Autodesk Inventor part; units mm, degrees
(part 2 of 3)
  arc A17 (-11.8052, -4.5833) -> (-10.4532, -3.3962) centre (-11.8777, -3.1373) ccw
  arc A18 (-11.8052, -4.5833) -> (-10.4532, -3.3962) centre (-11.8777, -3.1373) ccw
  line L518 (-12.3915, -4.5833) -> (-11.8052, -4.5833)
  line L519 (-11.8052, -4.5833) -> (-12.3915, -4.5833)
  arc A19 (-13.2869, -3.5243) -> (-12.3915, -4.5833) centre (-12.3915, -3.6753) ccw
  arc A20 (-13.2869, -3.5243) -> (-12.3915, -4.5833) centre (-12.3915, -3.6753) ccw
  line L520 (10.764, -4.357) -> (10.8318, -4.3058)
  line L521 (10.8318, -4.3058) -> (10.764, -4.357)
  line L522 (10.6948, -4.4031) -> (10.764, -4.357)
  line L523 (10.764, -4.357) -> (10.6948, -4.4031)
  line L524 (10.6242, -4.4442) -> (10.6948, -4.4031)
  line L525 (10.6948, -4.4031) -> (10.6242, -4.4442)
  line L526 (10.5766, -4.468) -> (10.6242, -4.4442)
  line L527 (10.6242, -4.4442) -> (10.5766, -4.468)
  line L528 (10.4995, -4.5019) -> (10.5766, -4.468)
  line L529 (10.5766, -4.468) -> (10.4995, -4.5019)
  line L530 (10.4201, -4.5314) -> (10.4995, -4.5019)
  line L531 (10.4995, -4.5019) -> (10.4201, -4.5314)
  line L532 (10.3401, -4.5552) -> (10.4201, -4.5314)
  line L533 (10.4201, -4.5314) -> (10.3401, -4.5552)
  line L534 (10.2587, -4.574) -> (10.3401, -4.5552)
  line L535 (10.3401, -4.5552) -> (10.2587, -4.574)
  line L536 (10.1757, -4.5877) -> (10.2587, -4.574)
  line L537 (10.2587, -4.574) -> (10.1757, -4.5877)
  line L538 (10.0914, -4.5956) -> (10.1757, -4.5877)
  line L539 (10.1757, -4.5877) -> (10.0914, -4.5956)
  line L540 (10.0063, -4.5985) -> (10.0914, -4.5956)
  line L541 (10.0914, -4.5956) -> (10.0063, -4.5985)
  line L542 (9.9984, -4.5985) -> (10.0063, -4.5985)
  line L543 (10.0063, -4.5985) -> (9.9984, -4.5985)
  line L544 (9.9112, -4.5956) -> (9.9984, -4.5985)
  line L545 (9.9984, -4.5985) -> (9.9112, -4.5956)
  line L546 (9.8261, -4.5869) -> (9.9112, -4.5956)
  line L547 (9.9112, -4.5956) -> (9.8261, -4.5869)
  line L548 (9.7432, -4.5725) -> (9.8261, -4.5869)
  line L549 (9.8261, -4.5869) -> (9.7432, -4.5725)
  line L550 (9.6631, -4.5523) -> (9.7432, -4.5725)
  line L551 (9.7432, -4.5725) -> (9.6631, -4.5523)
  line L552 (9.5846, -4.5257) -> (9.6631, -4.5523)
  line L553 (9.6631, -4.5523) -> (9.5846, -4.5257)
  line L554 (9.5081, -4.4939) -> (9.5846, -4.5257)
  line L555 (9.5846, -4.5257) -> (9.5081, -4.4939)
  line L556 (9.4346, -4.4557) -> (9.5081, -4.4939)
  line L557 (9.5081, -4.4939) -> (9.4346, -4.4557)
  line L558 (9.4173, -4.4464) -> (9.4346, -4.4557)
  line L559 (9.4346, -4.4557) -> (9.4173, -4.4464)
  line L560 (9.3452, -4.4002) -> (9.4173, -4.4464)
  line L561 (9.4173, -4.4464) -> (9.3452, -4.4002)
  line L562 (9.2782, -4.3498) -> (9.3452, -4.4002)
  line L563 (9.3452, -4.4002) -> (9.2782, -4.3498)
  line L564 (9.2169, -4.2942) -> (9.2782, -4.3498)
  line L565 (9.2782, -4.3498) -> (9.2169, -4.2942)
  line L566 (9.1599, -4.2344) -> (9.2169, -4.2942)
  line L567 (9.2169, -4.2942) -> (9.1599, -4.2344)
  line L568 (9.1087, -4.1688) -> (9.1599, -4.2344)
  line L569 (9.1599, -4.2344) -> (9.1087, -4.1688)
  line L570 (9.0626, -4.0989) -> (9.1087, -4.1688)
  line L571 (9.1087, -4.1688) -> (9.0626, -4.0989)
  line L572 (9.0215, -4.0239) -> (9.0626, -4.0989)
  line L573 (9.0626, -4.0989) -> (9.0215, -4.0239)
  line L574 (9.0186, -4.0188) -> (9.0215, -4.0239)
  line L575 (9.0215, -4.0239) -> (9.0186, -4.0188)
  line L576 (8.9833, -3.9417) -> (9.0186, -4.0188)
  line L577 (9.0186, -4.0188) -> (8.9833, -3.9417)
  line L578 (8.953, -3.8631) -> (8.9833, -3.9417)
  line L579 (8.9833, -3.9417) -> (8.953, -3.8631)
  line L580 (8.9285, -3.7831) -> (8.953, -3.8631)
  line L581 (8.953, -3.8631) -> (8.9285, -3.7831)
  line L582 (8.909, -3.7023) -> (8.9285, -3.7831)
  line L583 (8.9285, -3.7831) -> (8.909, -3.7023)
  line L584 (8.8946, -3.6194) -> (8.909, -3.7023)
  line L585 (8.909, -3.7023) -> (8.8946, -3.6194)
  line L586 (8.886, -3.5351) -> (8.8946, -3.6194)
  line L587 (8.8946, -3.6194) -> (8.886, -3.5351)
  line L588 (8.8824, -3.45) -> (8.886, -3.5351)
  line L589 (8.886, -3.5351) -> (8.8824, -3.45)
  line L590 (8.8824, -3.4363) -> (8.8824, -3.45)
  line L591 (8.8824, -3.45) -> (8.8824, -3.4363)
  line L592 (8.8845, -3.3433) -> (8.8824, -3.4363)
  line L593 (8.8824, -3.4363) -> (8.8845, -3.3433)
  line L594 (8.8896, -3.2525) -> (8.8845, -3.3433)
  line L595 (8.8845, -3.3433) -> (8.8896, -3.2525)
  line L596 (8.8989, -3.1645) -> (8.8896, -3.2525)
  line L597 (8.8896, -3.2525) -> (8.8989, -3.1645)
  line L598 (8.9112, -3.0787) -> (8.8989, -3.1645)
  line L599 (8.8989, -3.1645) -> (8.9112, -3.0787)
  line L600 (8.9278, -2.9951) -> (8.9112, -3.0787)
  line L601 (8.9112, -3.0787) -> (8.9278, -2.9951)
  line L602 (8.9472, -2.9136) -> (8.9278, -2.9951)
  line L603 (8.9278, -2.9951) -> (8.9472, -2.9136)
  line L604 (8.971, -2.8343) -> (8.9472, -2.9136)
  line L605 (8.9472, -2.9136) -> (8.971, -2.8343)
  line L606 (8.9977, -2.7579) -> (8.971, -2.8343)
  line L607 (8.971, -2.8343) -> (8.9977, -2.7579)
  line L608 (9.0287, -2.6843) -> (8.9977, -2.7579)
  line L609 (8.9977, -2.7579) -> (9.0287, -2.6843)
  line L610 (9.0626, -2.6122) -> (9.0287, -2.6843)
  line L611 (9.0287, -2.6843) -> (9.0626, -2.6122)
  line L612 (9.1008, -2.543) -> (9.0626, -2.6122)
  line L613 (9.0626, -2.6122) -> (9.1008, -2.543)
  line L614 (9.1419, -2.476) -> (9.1008, -2.543)
  line L615 (9.1008, -2.543) -> (9.1419, -2.476)
  line L616 (9.1873, -2.4111) -> (9.1419, -2.476)
  line L617 (9.1419, -2.476) -> (9.1873, -2.4111)
  line L618 (9.2363, -2.3491) -> (9.1873, -2.4111)
  line L619 (9.1873, -2.4111) -> (9.2363, -2.3491)
  line L620 (9.2882, -2.2893) -> (9.2363, -2.3491)
  line L621 (9.2363, -2.3491) -> (9.2882, -2.2893)
  line L622 (9.2955, -2.2813) -> (9.2882, -2.2893)
  line L623 (9.2882, -2.2893) -> (9.2955, -2.2813)
  line L624 (9.3567, -2.2193) -> (9.2955, -2.2813)
  line L625 (9.2955, -2.2813) -> (9.3567, -2.2193)
  line L626 (9.4202, -2.1617) -> (9.3567, -2.2193)
  line L627 (9.3567, -2.2193) -> (9.4202, -2.1617)
  line L628 (9.4851, -2.109) -> (9.4202, -2.1617)
  line L629 (9.4202, -2.1617) -> (9.4851, -2.109)
  line L630 (9.5521, -2.0607) -> (9.4851, -2.109)
  line L631 (9.4851, -2.109) -> (9.5521, -2.0607)
  line L632 (9.6213, -2.0175) -> (9.5521, -2.0607)
  line L633 (9.5521, -2.0607) -> (9.6213, -2.0175)
  line L634 (9.692, -1.9785) -> (9.6213, -2.0175)
  line L635 (9.6213, -2.0175) -> (9.692, -1.9785)
  line L636 (9.7648, -1.9446) -> (9.692, -1.9785)
  line L637 (9.692, -1.9785) -> (9.7648, -1.9446)
  line L638 (9.8398, -1.9158) -> (9.7648, -1.9446)
  line L639 (9.7648, -1.9446) -> (9.8398, -1.9158)
  line L640 (9.9162, -1.8913) -> (9.8398, -1.9158)
  line L641 (9.8398, -1.9158) -> (9.9162, -1.8913)
  line L642 (9.9948, -1.8718) -> (9.9162, -1.8913)
  line L643 (9.9162, -1.8913) -> (9.9948, -1.8718)
  line L644 (10.0755, -1.8574) -> (9.9948, -1.8718)
  line L645 (9.9948, -1.8718) -> (10.0755, -1.8574)
  line L646 (10.1577, -1.8473) -> (10.0755, -1.8574)
  line L647 (10.0755, -1.8574) -> (10.1577, -1.8473)
  line L648 (10.2421, -1.8423) -> (10.1577, -1.8473)
  line L649 (10.1577, -1.8473) -> (10.2421, -1.8423)
  line L650 (10.2933, -1.8415) -> (10.2421, -1.8423)
  line L651 (10.2421, -1.8423) -> (10.2933, -1.8415)
  line L652 (10.3834, -1.8444) -> (10.2933, -1.8415)
  line L653 (10.2933, -1.8415) -> (10.3834, -1.8444)
  line L654 (10.4706, -1.8524) -> (10.3834, -1.8444)
  line L655 (10.3834, -1.8444) -> (10.4706, -1.8524)
  line L656 (10.5542, -1.8661) -> (10.4706, -1.8524)
  line L657 (10.4706, -1.8524) -> (10.5542, -1.8661)
  line L658 (10.635, -1.8855) -> (10.5542, -1.8661)
  line L659 (10.5542, -1.8661) -> (10.635, -1.8855)
  line L660 (10.7129, -1.91) -> (10.635, -1.8855)
  line L661 (10.635, -1.8855) -> (10.7129, -1.91)
  line L662 (10.7871, -1.9403) -> (10.7129, -1.91)
  line L663 (10.7129, -1.91) -> (10.7871, -1.9403)
  line L664 (10.8585, -1.9756) -> (10.7871, -1.9403)
  line L665 (10.7871, -1.9403) -> (10.8585, -1.9756)
  line L666 (10.927, -2.0167) -> (10.8585, -1.9756)
  line L667 (10.8585, -1.9756) -> (10.927, -2.0167)
  line L668 (10.9926, -2.0636) -> (10.927, -2.0167)
  line L669 (10.927, -2.0167) -> (10.9926, -2.0636)
  line L670 (11.0546, -2.1155) -> (10.9926, -2.0636)
  line L671 (10.9926, -2.0636) -> (11.0546, -2.1155)
  line L672 (11.1058, -2.1653) -> (11.0546, -2.1155)
  line L673 (11.0546, -2.1155) -> (11.1058, -2.1653)
  line L674 (11.1584, -2.2237) -> (11.1058, -2.1653)
  line L675 (11.1058, -2.1653) -> (11.1584, -2.2237)
  line L676 (11.206, -2.2857) -> (11.1584, -2.2237)
  line L677 (11.1584, -2.2237) -> (11.206, -2.2857)
  line L678 (11.2485, -2.3513) -> (11.206, -2.2857)
  line L679 (11.206, -2.2857) -> (11.2485, -2.3513)
  line L680 (11.286, -2.4198) -> (11.2485, -2.3513)
  line L681 (11.2485, -2.3513) -> (11.286, -2.4198)
  line L682 (11.3192, -2.4918) -> (11.286, -2.4198)
  line L683 (11.286, -2.4198) -> (11.3192, -2.4918)
  line L684 (11.348, -2.5675) -> (11.3192, -2.4918)
  line L685 (11.3192, -2.4918) -> (11.348, -2.5675)
  line L686 (11.3718, -2.6461) -> (11.348, -2.5675)
  line L687 (11.348, -2.5675) -> (11.3718, -2.6461)
  line L688 (11.3906, -2.7283) -> (11.3718, -2.6461)
  line L689 (11.3718, -2.6461) -> (11.3906, -2.7283)
  line L690 (11.4043, -2.8141) -> (11.3906, -2.7283)
  line L691 (11.3906, -2.7283) -> (11.4043, -2.8141)
  line L692 (11.4136, -2.9028) -> (11.4043, -2.8141)
  line L693 (11.4043, -2.8141) -> (11.4136, -2.9028)
  line L694 (11.418, -2.9951) -> (11.4136, -2.9028)
  line L695 (11.4136, -2.9028) -> (11.418, -2.9951)
  line L696 (11.4187, -3.0362) -> (11.418, -2.9951)
  line L697 (11.418, -2.9951) -> (11.4187, -3.0362)
  line L698 (11.4165, -3.1241) -> (11.4187, -3.0362)
  line L699 (11.4187, -3.0362) -> (11.4165, -3.1241)
  line L700 (11.4107, -3.2099) -> (11.4165, -3.1241)
  line L701 (11.4165, -3.1241) -> (11.4107, -3.2099)
  line L702 (11.3999, -3.2943) -> (11.4107, -3.2099)
  line L703 (11.4107, -3.2099) -> (11.3999, -3.2943)
  line L704 (11.3862, -3.3772) -> (11.3999, -3.2943)
  line L705 (11.3999, -3.2943) -> (11.3862, -3.3772)
  line L706 (11.3675, -3.4594) -> (11.3862, -3.3772)
  line L707 (11.3862, -3.3772) -> (11.3675, -3.4594)
  line L708 (11.3459, -3.5394) -> (11.3675, -3.4594)
  line L709 (11.3675, -3.4594) -> (11.3459, -3.5394)
  line L710 (11.3192, -3.618) -> (11.3459, -3.5394)
  line L711 (11.3459, -3.5394) -> (11.3192, -3.618)
  line L712 (11.2889, -3.6951) -> (11.3192, -3.618)
  line L713 (11.3192, -3.618) -> (11.2889, -3.6951)
  line L714 (11.2601, -3.7586) -> (11.2889, -3.6951)
  line L715 (11.2889, -3.6951) -> (11.2601, -3.7586)
  line L716 (11.2204, -3.8372) -> (11.2601, -3.7586)
  line L717 (11.2601, -3.7586) -> (11.2204, -3.8372)
  line L718 (11.1779, -3.9121) -> (11.2204, -3.8372)
  line L719 (11.2204, -3.8372) -> (11.1779, -3.9121)
  line L720 (11.1317, -3.9835) -> (11.1779, -3.9121)
  line L721 (11.1779, -3.9121) -> (11.1317, -3.9835)
  line L722 (11.082, -4.0513) -> (11.1317, -3.9835)
  line L723 (11.1317, -3.9835) -> (11.082, -4.0513)
  line L724 (11.0294, -4.1154) -> (11.082, -4.0513)
  line L725 (11.082, -4.0513) -> (11.0294, -4.1154)
  line L726 (10.9738, -4.176) -> (11.0294, -4.1154)
  line L727 (11.0294, -4.1154) -> (10.9738, -4.176)
  line L728 (10.9623, -4.1875) -> (10.9738, -4.176)
  line L729 (10.9738, -4.176) -> (10.9623, -4.1875)
  line L730 (10.8974, -4.2495) -> (10.9623, -4.1875)
  line L731 (10.9623, -4.1875) -> (10.8974, -4.2495)
  line L732 (10.8318, -4.3058) -> (10.8974, -4.2495)
  line L733 (10.8974, -4.2495) -> (10.8318, -4.3058)
  line L734 (-3.4143, -2.0689) -> (-3.8594, -4.5927)
  line L735 (-3.8594, -4.5927) -> (-3.4143, -2.0689)
  line L736 (-1.6963, -2.0689) -> (-3.4143, -2.0689)
  line L737 (-3.4143, -2.0689) -> (-1.6963, -2.0689)
  arc A21 (-1.4506, -3.3546) -> (-1.6963, -2.0689) centre (-1.726, -2.7409) ccw
  arc A22 (-1.4506, -3.3546) -> (-1.6963, -2.0689) centre (-1.726, -2.7409) ccw
  arc A23 (-1.2403, -3.7043) -> (-1.4506, -3.3546) centre (-2.0068, -3.9272) ccw
  arc A24 (-1.2403, -3.7043) -> (-1.4506, -3.3546) centre (-2.0068, -3.9272) ccw
  line L738 (-1.0022, -4.5927) -> (-1.2403, -3.7043)
  line L739 (-1.2403, -3.7043) -> (-1.0022, -4.5927)
  line L740 (-1.7842, -4.5927) -> (-1.0022, -4.5927)
  line L741 (-1.0022, -4.5927) -> (-1.7842, -4.5927)
  line L742 (-1.9465, -3.9869) -> (-1.7842, -4.5927)
  line L743 (-1.7842, -4.5927) -> (-1.9465, -3.9869)
  arc A25 (-1.9465, -3.9869) -> (-2.544, -3.5591) centre (-2.5929, -4.2585) ccw
  arc A26 (-1.9465, -3.9869) -> (-2.544, -3.5591) centre (-2.5929, -4.2585) ccw
  line L744 (-2.8935, -3.5591) -> (-2.544, -3.5591)
  line L745 (-2.544, -3.5591) -> (-2.8935, -3.5591)
  line L746 (-3.0757, -4.5927) -> (-2.8935, -3.5591)
  line L747 (-2.8935, -3.5591) -> (-3.0757, -4.5927)
  line L748 (-3.8594, -4.5927) -> (-3.0757, -4.5927)
  line L749 (-3.0757, -4.5927) -> (-3.8594, -4.5927)
  line L750 (-9.2507, -2.0595) -> (-10.0381, -2.0595)
  line L751 (-10.0381, -2.0595) -> (-9.2507, -2.0595)
  line L752 (-9.134, -3.7743) -> (-9.2507, -2.0595)
  line L753 (-9.2507, -2.0595) -> (-9.134, -3.7743)
  line L754 (-8.4342, -2.0595) -> (-9.134, -3.7743)
  spline S0 degree 3 poles (0.7832, -2.4934) (0.8407, -2.4926) (0.8976, -2.5061) (1.0487, -2.5614) (1.1497, -2.6172) (1.3156, -2.7342) (1.3817, -2.7882) (1.4417, -2.8447) knots 4.484634 4.484634 4.484634 4.484634 4.865969 4.865969 5.478673 5.478673 5.90022 5.90022 5.90022 5.90022
  line L755 (0.7832, -2.4934) -> (0.8407, -2.4926) construction
  line L756 (0.8407, -2.4926) -> (0.8976, -2.5061) construction
  line L757 (0.8976, -2.5061) -> (1.0487, -2.5614) construction
  line L758 (1.0487, -2.5614) -> (1.1497, -2.6172) construction
  line L759 (1.1497, -2.6172) -> (1.3156, -2.7342) construction
  line L760 (1.3156, -2.7342) -> (1.3817, -2.7882) construction
  line L761 (1.3817, -2.7882) -> (1.4417, -2.8447) construction
  line L762 (-9.134, -3.7743) -> (-8.4342, -2.0595)
  spline S1 degree 3 poles (1.4417, -2.8447) (1.3817, -2.7882) (1.3156, -2.7342) (1.1497, -2.6172) (1.0487, -2.5614) (0.8976, -2.5061) (0.8407, -2.4926) (0.7832, -2.4934) knots -5.90022 -5.90022 -5.90022 -5.90022 -5.478673 -5.478673 -4.865969 -4.865969 -4.484634 -4.484634 -4.484634 -4.484634
  line L763 (1.4417, -2.8447) -> (1.3817, -2.7882) construction
  line L764 (1.3817, -2.7882) -> (1.3156, -2.7342) construction
  line L765 (1.3156, -2.7342) -> (1.1497, -2.6172) construction
  line L766 (1.1497, -2.6172) -> (1.0487, -2.5614) construction
  line L767 (1.0487, -2.5614) -> (0.8976, -2.5061) construction
  line L768 (0.8976, -2.5061) -> (0.8407, -2.4926) construction
  line L769 (0.8407, -2.4926) -> (0.7832, -2.4934) construction
  line L770 (-8.0608, -2.0595) -> (-8.4342, -2.0595)
  line L771 (-8.4342, -2.0595) -> (-8.0608, -2.0595)
  line L772 (-7.8698, -3.7104) -> (-8.0608, -2.0595)
  line L773 (-8.0608, -2.0595) -> (-7.8698, -3.7104)
  line L774 (-7.1961, -2.0595) -> (-7.8698, -3.7104)
  line L775 (-7.8698, -3.7104) -> (-7.1961, -2.0595)
  line L776 (-6.4191, -2.0595) -> (-7.1961, -2.0595)
  line L777 (-7.1961, -2.0595) -> (-6.4191, -2.0595)
  line L778 (-7.7213, -4.5833) -> (-6.4191, -2.0595)
  line L779 (-6.4191, -2.0595) -> (-7.7213, -4.5833)
  line L780 (-8.1744, -4.5833) -> (-7.7213, -4.5833)
  line L781 (-7.7213, -4.5833) -> (-8.1744, -4.5833)
  line L782 (-8.4008, -2.9217) -> (-8.1744, -4.5833)
  line L783 (-8.1744, -4.5833) -> (-8.4008, -2.9217)
  line L784 (-9.1859, -4.5833) -> (-8.4008, -2.9217)
  line L785 (-8.4008, -2.9217) -> (-9.1859, -4.5833)
  line L786 (-9.626, -4.5833) -> (-9.1859, -4.5833)
  line L787 (-9.1859, -4.5833) -> (-9.626, -4.5833)
  line L788 (-10.0381, -2.0595) -> (-9.626, -4.5833)
  line L789 (-9.626, -4.5833) -> (-10.0381, -2.0595)
  line L790 (6.6315, -3.3693) -> (7.0461, -3.3693)
  line L791 (7.0461, -3.3693) -> (6.6315, -3.3693)
  line L792 (6.385, -4.5531) -> (6.6315, -3.3693)
  line L793 (6.6315, -3.3693) -> (6.385, -4.5531)
  line L794 (6.0281, -4.5531) -> (6.385, -4.5531)
  line L795 (6.385, -4.5531) -> (6.0281, -4.5531)
  line L796 (6.5861, -1.887) -> (6.0281, -4.5531)
  line L797 (6.0281, -4.5531) -> (6.5861, -1.887)
  line L798 (7.7043, -1.887) -> (6.5861, -1.887)
  line L799 (6.5861, -1.887) -> (7.7043, -1.887)
  line L800 (7.811, -1.8884) -> (7.7043, -1.887)
  line L801 (7.7043, -1.887) -> (7.811, -1.8884)
  line L802 (7.9083, -1.8927) -> (7.811, -1.8884)
  line L803 (7.811, -1.8884) -> (7.9083, -1.8927)
  line L804 (7.9963, -1.9007) -> (7.9083, -1.8927)
  line L805 (7.9083, -1.8927) -> (7.9963, -1.9007)
  line L806 (8.0756, -1.9115) -> (7.9963, -1.9007)
  line L807 (7.9963, -1.9007) -> (8.0756, -1.9115)
  line L808 (8.1463, -1.9252) -> (8.0756, -1.9115)
  line L809 (8.0756, -1.9115) -> (8.1463, -1.9252)
  line L810 (8.2061, -1.941) -> (8.1463, -1.9252)
  line L811 (8.1463, -1.9252) -> (8.2061, -1.941)
  line L812 (8.284, -1.9742) -> (8.2061, -1.941)
  line L813 (8.2061, -1.941) -> (8.284, -1.9742)
  line L814 (8.3532, -2.0175) -> (8.284, -1.9742)
  line L815 (8.284, -1.9742) -> (8.3532, -2.0175)
  line L816 (8.4145, -2.0723) -> (8.3532, -2.0175)
  line L817 (8.3532, -2.0175) -> (8.4145, -2.0723)
  line L818 (8.4671, -2.1386) -> (8.4145, -2.0723)
  line L819 (8.4145, -2.0723) -> (8.4671, -2.1386)
  line L820 (8.475, -2.1508) -> (8.4671, -2.1386)
  line L821 (8.4671, -2.1386) -> (8.475, -2.1508)
  line L822 (8.5111, -2.2179) -> (8.475, -2.1508)
  line L823 (8.475, -2.1508) -> (8.5111, -2.2179)
  line L824 (8.5392, -2.2921) -> (8.5111, -2.2179)
  line L825 (8.5111, -2.2179) -> (8.5392, -2.2921)
  line L826 (8.5579, -2.3729) -> (8.5392, -2.2921)
  line L827 (8.5392, -2.2921) -> (8.5579, -2.3729)
  line L828 (8.5687, -2.4608) -> (8.5579, -2.3729)
  line L829 (8.5579, -2.3729) -> (8.5687, -2.4608)
  line L830 (8.5716, -2.5358) -> (8.5687, -2.4608)
  line L831 (8.5687, -2.4608) -> (8.5716, -2.5358)
  line L832 (8.5673, -2.6245) -> (8.5716, -2.5358)
  line L833 (8.5716, -2.5358) -> (8.5673, -2.6245)
  line L834 (8.555, -2.7089) -> (8.5673, -2.6245)
  line L835 (8.5673, -2.6245) -> (8.555, -2.7089)
  line L836 (8.5349, -2.7882) -> (8.555, -2.7089)
  line L837 (8.555, -2.7089) -> (8.5349, -2.7882)
  line L838 (8.506, -2.8639) -> (8.5349, -2.7882)
  line L839 (8.5349, -2.7882) -> (8.506, -2.8639)
  line L840 (8.4685, -2.9352) -> (8.506, -2.8639)
  line L841 (8.506, -2.8639) -> (8.4685, -2.9352)
  line L842 (8.4238, -3.0023) -> (8.4685, -2.9352)
  line L843 (8.4685, -2.9352) -> (8.4238, -3.0023)
  line L844 (8.3698, -3.065) -> (8.4238, -3.0023)
  line L845 (8.4238, -3.0023) -> (8.3698, -3.065)
  line L846 (8.3589, -3.0765) -> (8.3698, -3.065)
  line L847 (8.3698, -3.065) -> (8.3589, -3.0765)
  line L848 (8.3085, -3.122) -> (8.3589, -3.0765)
  line L849 (8.3589, -3.0765) -> (8.3085, -3.122)
  line L850 (8.2515, -3.1638) -> (8.3085, -3.122)
  line L851 (8.3085, -3.122) -> (8.2515, -3.1638)
  line L852 (8.1888, -3.2027) -> (8.2515, -3.1638)
  line L853 (8.2515, -3.1638) -> (8.1888, -3.2027)
  line L854 (8.1189, -3.2373) -> (8.1888, -3.2027)
  line L855 (8.1888, -3.2027) -> (8.1189, -3.2373)
  line L856 (8.0432, -3.2676) -> (8.1189, -3.2373)
  line L857 (8.1189, -3.2373) -> (8.0432, -3.2676)
  line L858 (7.9602, -3.295) -> (8.0432, -3.2676)
  line L859 (8.0432, -3.2676) -> (7.9602, -3.295)
  line L860 (7.8716, -3.3188) -> (7.9602, -3.295)
  line L861 (7.9602, -3.295) -> (7.8716, -3.3188)
  line L862 (7.7764, -3.3383) -> (7.8716, -3.3188)
  line L863 (7.8716, -3.3188) -> (7.7764, -3.3383)
  line L864 (7.674, -3.3541) -> (7.7764, -3.3383)
  line L865 (7.7764, -3.3383) -> (7.674, -3.3541)
  line L866 (7.6719, -3.3548) -> (7.674, -3.3541)
  line L867 (7.674, -3.3541) -> (7.6719, -3.3548)
  line L868 (7.7468, -3.414) -> (7.6719, -3.3548)
  line L869 (7.6719, -3.3548) -> (7.7468, -3.414)
  line L870 (7.811, -3.4723) -> (7.7468, -3.414)
  line L871 (7.7468, -3.414) -> (7.811, -3.4723)
  line L872 (7.8644, -3.5307) -> (7.811, -3.4723)
  line L873 (7.811, -3.4723) -> (7.8644, -3.5307)
  line L874 (7.8918, -3.5654) -> (7.8644, -3.5307)
  line L875 (7.8644, -3.5307) -> (7.8918, -3.5654)
  line L876 (7.9415, -3.6374) -> (7.8918, -3.5654)
  line L877 (7.8918, -3.5654) -> (7.9415, -3.6374)
  line L878 (7.9876, -3.7103) -> (7.9415, -3.6374)
  line L879 (7.9415, -3.6374) -> (7.9876, -3.7103)
  line L880 (8.0309, -3.7838) -> (7.9876, -3.7103)
  line L881 (7.9876, -3.7103) -> (8.0309, -3.7838)
  line L882 (8.0713, -3.8581) -> (8.0309, -3.7838)
  line L883 (8.0309, -3.7838) -> (8.0713, -3.8581)
  line L884 (8.1088, -3.933) -> (8.0713, -3.8581)
  line L885 (8.0713, -3.8581) -> (8.1088, -3.933)
  line L886 (8.1434, -4.0087) -> (8.1088, -3.933)
  line L887 (8.1088, -3.933) -> (8.1434, -4.0087)
  line L888 (8.1607, -4.0513) -> (8.1434, -4.0087)
  line L889 (8.1434, -4.0087) -> (8.1607, -4.0513)
  line L890 (8.3647, -4.5531) -> (8.1607, -4.0513)
  line L891 (8.1607, -4.0513) -> (8.3647, -4.5531)
  line L892 (7.966, -4.5531) -> (8.3647, -4.5531)
  line L893 (8.3647, -4.5531) -> (7.966, -4.5531)
  line L894 (7.7757, -4.057) -> (7.966, -4.5531)
  line L895 (7.966, -4.5531) -> (7.7757, -4.057)
  line L896 (7.7411, -3.9712) -> (7.7757, -4.057)
  line L897 (7.7757, -4.057) -> (7.7411, -3.9712)
  line L898 (7.705, -3.8898) -> (7.7411, -3.9712)
  line L899 (7.7411, -3.9712) -> (7.705, -3.8898)
  line L900 (7.6675, -3.8119) -> (7.705, -3.8898)
  line L901 (7.705, -3.8898) -> (7.6675, -3.8119)
  line L902 (7.6286, -3.7377) -> (7.6675, -3.8119)
  line L903 (7.6675, -3.8119) -> (7.6286, -3.7377)
  line L904 (7.5882, -3.6677) -> (7.6286, -3.7377)
  line L905 (7.6286, -3.7377) -> (7.5882, -3.6677)
  line L906 (7.5457, -3.6014) -> (7.5882, -3.6677)
  line L907 (7.5882, -3.6677) -> (7.5457, -3.6014)
  line L908 (7.5392, -3.5913) -> (7.5457, -3.6014)
  line L909 (7.5457, -3.6014) -> (7.5392, -3.5913)
  line L910 (7.4801, -3.5127) -> (7.5392, -3.5913)
  line L911 (7.5392, -3.5913) -> (7.4801, -3.5127)
  line L912 (7.421, -3.4543) -> (7.4801, -3.5127)
  line L913 (7.4801, -3.5127) -> (7.421, -3.4543)
  line L914 (7.3604, -3.4147) -> (7.421, -3.4543)
  line L915 (7.421, -3.4543) -> (7.3604, -3.4147)
  line L916 (7.3539, -3.4111) -> (7.3604, -3.4147)
  line L917 (7.3604, -3.4147) -> (7.3539, -3.4111)
  line L918 (7.2934, -3.3916) -> (7.3539, -3.4111)
  line L919 (7.3539, -3.4111) -> (7.2934, -3.3916)
  line L920 (7.2162, -3.3779) -> (7.2934, -3.3916)
  line L921 (7.2934, -3.3916) -> (7.2162, -3.3779)
  line L922 (7.1218, -3.3707) -> (7.2162, -3.3779)
  line L923 (7.2162, -3.3779) -> (7.1218, -3.3707)
  line L924 (7.0461, -3.3693) -> (7.1218, -3.3707)
  line L925 (7.1218, -3.3707) -> (7.0461, -3.3693)
  line L926 (-3.9191, -2.0689) -> (-5.9191, -2.0689)
  line L927 (-5.9191, -2.0689) -> (-3.9191, -2.0689)
  line L928 (-3.994, -2.4934) -> (-3.9191, -2.0689)
  line L929 (-3.9191, -2.0689) -> (-3.994, -2.4934)
  line L930 (-5.202, -2.4934) -> (-3.994, -2.4934)
  line L931 (-3.994, -2.4934) -> (-5.202, -2.4934)
  line L932 (-5.3149, -3.1336) -> (-5.202, -2.4934)
  line L933 (-5.202, -2.4934) -> (-5.3149, -3.1336)
  line L934 (-4.2021, -3.1336) -> (-5.3149, -3.1336)
  line L935 (-5.3149, -3.1336) -> (-4.2021, -3.1336)
  line L936 (-4.2717, -3.5281) -> (-4.2021, -3.1336)
  line L937 (-4.2021, -3.1336) -> (-4.2717, -3.5281)
  line L938 (-5.3845, -3.5281) -> (-4.2717, -3.5281)
  line L939 (-4.2717, -3.5281) -> (-5.3845, -3.5281)
  line L940 (-5.4974, -4.1682) -> (-5.3845, -3.5281)
  line L941 (-5.3845, -3.5281) -> (-5.4974, -4.1682)
  line L942 (-4.2893, -4.1682) -> (-5.4974, -4.1682)
  line L943 (-5.4974, -4.1682) -> (-4.2893, -4.1682)
  line L944 (-4.3642, -4.5927) -> (-4.2893, -4.1682)
  line L945 (-4.2893, -4.1682) -> (-4.3642, -4.5927)
  line L946 (-6.3642, -4.5927) -> (-4.3642, -4.5927)
  line L947 (-4.3642, -4.5927) -> (-6.3642, -4.5927)
  line L948 (-5.9191, -2.0689) -> (-6.3642, -4.5927)
  line L949 (-6.3642, -4.5927) -> (-5.9191, -2.0689)
  line L950 (16.3572, -3.2784) -> (16.4235, -3.2243)
  line L951 (16.4235, -3.2243) -> (16.3572, -3.2784)
  line L952 (16.2916, -3.3209) -> (16.3572, -3.2784)
  line L953 (16.3572, -3.2784) -> (16.2916, -3.3209)
  line L954 (16.2801, -3.3274) -> (16.2916, -3.3209)
  line L955 (16.2916, -3.3209) -> (16.2801, -3.3274)
  line L956 (16.2037, -3.3635) -> (16.2801, -3.3274)
  line L957 (16.2801, -3.3274) -> (16.2037, -3.3635)
  line L958 (16.1243, -3.3923) -> (16.2037, -3.3635)
  line L959 (16.2037, -3.3635) -> (16.1243, -3.3923)
  line L960 (16.0544, -3.4111) -> (16.1243, -3.3923)
  line L961 (16.1243, -3.3923) -> (16.0544, -3.4111)
  line L962 (15.9708, -3.4291) -> (16.0544, -3.4111)
  line L963 (16.0544, -3.4111) -> (15.9708, -3.4291)
  line L964 (15.8872, -3.4435) -> (15.9708, -3.4291)
  line L965 (15.9708, -3.4291) -> (15.8872, -3.4435)
  line L966 (15.8035, -3.455) -> (15.8872, -3.4435)
  line L967 (15.8872, -3.4435) -> (15.8035, -3.455)
  line L968 (15.7192, -3.4637) -> (15.8035, -3.455)
  line L969 (15.8035, -3.455) -> (15.7192, -3.4637)
  line L970 (15.6348, -3.4687) -> (15.7192, -3.4637)
  line L971 (15.7192, -3.4637) -> (15.6348, -3.4687)
  line L972 (15.5497, -3.4709) -> (15.6348, -3.4687)
  line L973 (15.6348, -3.4687) -> (15.5497, -3.4709)
  line L974 (14.8692, -3.4709) -> (15.5497, -3.4709)
  line L975 (15.5497, -3.4709) -> (14.8692, -3.4709)
  line L976 (14.6435, -4.5531) -> (14.8692, -3.4709)
  line L977 (14.8692, -3.4709) -> (14.6435, -4.5531)
  line L978 (14.2874, -4.5531) -> (14.6435, -4.5531)
  line L979 (14.6435, -4.5531) -> (14.2874, -4.5531)
  line L980 (14.8454, -1.887) -> (14.2874, -4.5531)
  line L981 (14.2874, -4.5531) -> (14.8454, -1.887)
  line L982 (15.9578, -1.887) -> (14.8454, -1.887)
  line L983 (14.8454, -1.887) -> (15.9578, -1.887)
  line L984 (16.0631, -1.8891) -> (15.9578, -1.887)
  line L985 (15.9578, -1.887) -> (16.0631, -1.8891)
  line L986 (16.1575, -1.8963) -> (16.0631, -1.8891)
  line L987 (16.0631, -1.8891) -> (16.1575, -1.8963)
  line L988 (16.2419, -1.9086) -> (16.1575, -1.8963)
  line L989 (16.1575, -1.8963) -> (16.2419, -1.9086)
  line L990 (16.3154, -1.9252) -> (16.2419, -1.9086)
  line L991 (16.2419, -1.9086) -> (16.3154, -1.9252)
  line L992 (16.3788, -1.9468) -> (16.3154, -1.9252)
  line L993 (16.3154, -1.9252) -> (16.3788, -1.9468)
  line L994 (16.3925, -1.9526) -> (16.3788, -1.9468)
  line L995 (16.3788, -1.9468) -> (16.3925, -1.9526)
  line L996 (16.461, -1.9922) -> (16.3925, -1.9526)
  line L997 (16.3925, -1.9526) -> (16.461, -1.9922)
  line L998 (16.5245, -2.0434) -> (16.461, -1.9922)
  line L999 (16.461, -1.9922) -> (16.5245, -2.0434)
  line L1000 (16.5807, -2.1061) -> (16.5245, -2.0434)
  line L1001 (16.5245, -2.0434) -> (16.5807, -2.1061)
  line L1002 (16.6305, -2.1797) -> (16.5807, -2.1061)
  line L1003 (16.5807, -2.1061) -> (16.6305, -2.1797)
  line L1004 (16.6679, -2.2532) -> (16.6305, -2.1797)
  line L1005 (16.6305, -2.1797) -> (16.6679, -2.2532)
  line L1006 (16.6961, -2.3311) -> (16.6679, -2.2532)
  line L1007 (16.6679, -2.2532) -> (16.6961, -2.3311)
  line L1008 (16.7148, -2.4125) -> (16.6961, -2.3311)
  line L1009 (16.6961, -2.3311) -> (16.7148, -2.4125)
  line L1010 (16.7242, -2.4976) -> (16.7148, -2.4125)
  line L1011 (16.7148, -2.4125) -> (16.7242, -2.4976)
  line L1012 (16.7249, -2.5416) -> (16.7242, -2.4976)
  line L1013 (16.7242, -2.4976) -> (16.7249, -2.5416)
  line L1014 (16.7213, -2.6231) -> (16.7249, -2.5416)
  line L1015 (16.7249, -2.5416) -> (16.7213, -2.6231)
  line L1016 (16.709, -2.7053) -> (16.7213, -2.6231)
  line L1017 (16.7213, -2.6231) -> (16.709, -2.7053)
  line L1018 (16.6889, -2.7882) -> (16.709, -2.7053)
  line L1019 (16.709, -2.7053) -> (16.6889, -2.7882)
  line L1020 (16.6607, -2.8718) -> (16.6889, -2.7882)
  line L1021 (16.6889, -2.7882) -> (16.6607, -2.8718)
  line L1022 (16.6579, -2.8783) -> (16.6607, -2.8718)
  line L1023 (16.6607, -2.8718) -> (16.6579, -2.8783)
  line L1024 (16.6211, -2.9619) -> (16.6579, -2.8783)
  line L1025 (16.6579, -2.8783) -> (16.6211, -2.9619)
  line L1026 (16.58, -3.0376) -> (16.6211, -2.9619)
  line L1027 (16.6211, -2.9619) -> (16.58, -3.0376)
  line L1028 (16.5338, -3.1054) -> (16.58, -3.0376)
  line L1029 (16.58, -3.0376) -> (16.5338, -3.1054)
  line L1030 (16.4891, -3.1602) -> (16.5338, -3.1054)
  line L1031 (16.5338, -3.1054) -> (16.4891, -3.1602)
  line L1032 (16.4235, -3.2243) -> (16.4891, -3.1602)
  line L1033 (16.4891, -3.1602) -> (16.4235, -3.2243)
  line L1034 (0.1973, -4.5927) -> (0.6148, -4.5927)
  line L1035 (0.6148, -4.5927) -> (0.1973, -4.5927)
  arc A27 (-0.5477, -4.4051) -> (0.1973, -4.5927) centre (0.1995, -3.0111) ccw
  arc A28 (-0.5477, -4.4051) -> (0.1973, -4.5927) centre (0.1995, -3.0111) ccw
  line L1036 (-0.4491, -3.846) -> (-0.5477, -4.4051)
  line L1037 (-0.5477, -4.4051) -> (-0.4491, -3.846)
  arc A29 (-0.4491, -3.846) -> (0.221, -4.1475) centre (1.0231, -1.4694) ccw
  arc A30 (-0.4491, -3.846) -> (0.221, -4.1475) centre (1.0231, -1.4694) ccw
  spline S2 degree 3 poles (0.3525, -4.1684) (0.3082, -4.1688) (0.2647, -4.1605) (0.221, -4.1475) knots 5.607238 5.607238 5.607238 5.607238 5.899629 5.899629 5.899629 5.899629
  line L1038 (0.3525, -4.1684) -> (0.3082, -4.1688) construction
  line L1039 (0.3082, -4.1688) -> (0.2647, -4.1605) construction
  line L1040 (0.2647, -4.1605) -> (0.221, -4.1475) construction
  spline S3 degree 3 poles (0.221, -4.1475) (0.2647, -4.1605) (0.3082, -4.1688) (0.3525, -4.1684) knots -5.899629 -5.899629 -5.899629 -5.899629 -5.607238 -5.607238 -5.607238 -5.607238
  line L1041 (0.221, -4.1475) -> (0.2647, -4.1605) construction
  line L1042 (0.2647, -4.1605) -> (0.3082, -4.1688) construction
  line L1043 (0.3082, -4.1688) -> (0.3525, -4.1684) construction
  arc A31 (0.3525, -4.1684) -> (0.4849, -3.582) centre (0.3521, -3.8601) ccw
  arc A32 (0.3525, -4.1684) -> (0.4849, -3.582) centre (0.3521, -3.8601) ccw
  line L1044 (0.0726, -3.3754) -> (0.4849, -3.582)
  line L1045 (0.4849, -3.582) -> (0.0726, -3.3754)
  arc A33 (-0.2619, -2.715) -> (0.0726, -3.3754) centre (0.3342, -2.828) ccw
  arc A34 (-0.2619, -2.715) -> (0.0726, -3.3754) centre (0.3342, -2.828) ccw
  arc A35 (0.5213, -2.0689) -> (-0.2619, -2.715) centre (0.5213, -2.8666) ccw
  arc A36 (0.5213, -2.0689) -> (-0.2619, -2.715) centre (0.5213, -2.8666) ccw
  line L1046 (0.7868, -2.0689) -> (0.5213, -2.0689)
  line L1047 (0.5213, -2.0689) -> (0.7868, -2.0689)
  arc A37 (0.7935, -2.0689) -> (0.7868, -2.0689) centre (0.7982, -3.6505) ccw
  arc A38 (0.7935, -2.0689) -> (0.7868, -2.0689) centre (0.7982, -3.6505) ccw
  line L1048 (0.8097, -2.0689) -> (0.7935, -2.0689)
  line L1049 (0.7935, -2.0689) -> (0.8097, -2.0689)
  arc A39 (1.5455, -2.2565) -> (0.8097, -2.0689) centre (0.7982, -3.6505) ccw
  arc A40 (1.5455, -2.2565) -> (0.8097, -2.0689) centre (0.7982, -3.6505) ccw
  line L1050 (1.4417, -2.8447) -> (1.5455, -2.2565)
  line L1051 (1.5455, -2.2565) -> (1.4417, -2.8447)
  arc A41 (0.7832, -2.4934) -> (0.6511, -3.0796) centre (0.8036, -2.806) ccw
  arc A42 (0.7832, -2.4934) -> (0.6511, -3.0796) centre (0.8036, -2.806) ccw
  line L1052 (1.0669, -3.2879) -> (0.6511, -3.0796)
  line L1053 (0.6511, -3.0796) -> (1.0669, -3.2879)
  arc A43 (1.3891, -3.9863) -> (1.0669, -3.2879) centre (0.7759, -3.8457) ccw
  arc A44 (1.3891, -3.9863) -> (1.0669, -3.2879) centre (0.7759, -3.8457) ccw
  arc A45 (0.6148, -4.5927) -> (1.3891, -3.9863) centre (0.6148, -3.795) ccw
  arc A46 (0.6148, -4.5927) -> (1.3891, -3.9863) centre (0.6148, -3.795) ccw
  line L1054 (12.1908, -3.5257) -> (12.5333, -1.887)
  line L1055 (12.5333, -1.887) -> (12.1908, -3.5257)
  line L1056 (12.1713, -3.631) -> (12.1908, -3.5257)
  line L1057 (12.1908, -3.5257) -> (12.1713, -3.631)
  line L1058 (12.1577, -3.7196) -> (12.1713, -3.631)
  line L1059 (12.1713, -3.631) -> (12.1577, -3.7196)
  line L1060 (12.1504, -3.7925) -> (12.1577, -3.7196)
  line L1061 (12.1577, -3.7196) -> (12.1504, -3.7925)
  line L1062 (12.149, -3.8278) -> (12.1504, -3.7925)
  line L1063 (12.1504, -3.7925) -> (12.149, -3.8278)
  line L1064 (12.1562, -3.9121) -> (12.149, -3.8278)
  line L1065 (12.149, -3.8278) -> (12.1562, -3.9121)
  line L1066 (12.1778, -3.99) -> (12.1562, -3.9121)
  line L1067 (12.1562, -3.9121) -> (12.1778, -3.99)
  line L1068 (12.2139, -4.0606) -> (12.1778, -3.99)
  line L1069 (12.1778, -3.99) -> (12.2139, -4.0606)
  line L1070 (12.2636, -4.1241) -> (12.2139, -4.0606)
  line L1071 (12.2139, -4.0606) -> (12.2636, -4.1241)
  line L1072 (12.3184, -4.1731) -> (12.2636, -4.1241)
  line L1073 (12.2636, -4.1241) -> (12.3184, -4.1731)
  line L1074 (12.3833, -4.2171) -> (12.3184, -4.1731)
  line L1075 (12.3184, -4.1731) -> (12.3833, -4.2171)
  line L1076 (12.4547, -4.2517) -> (12.3833, -4.2171)
  line L1077 (12.3833, -4.2171) -> (12.4547, -4.2517)
  line L1078 (12.5318, -4.2777) -> (12.4547, -4.2517)
  line L1079 (12.4547, -4.2517) -> (12.5318, -4.2777)
  line L1080 (12.6147, -4.295) -> (12.5318, -4.2777)
  line L1081 (12.5318, -4.2777) -> (12.6147, -4.295)
  line L1082 (12.7041, -4.3036) -> (12.6147, -4.295)
  line L1083 (12.6147, -4.295) -> (12.7041, -4.3036)
  line L1084 (12.7438, -4.3043) -> (12.7041, -4.3036)
  line L1085 (12.7041, -4.3036) -> (12.7438, -4.3043)
  line L1086 (12.8296, -4.3) -> (12.7438, -4.3043)
  line L1087 (12.7438, -4.3043) -> (12.8296, -4.3)
  line L1088 (12.9125, -4.287) -> (12.8296, -4.3)
  line L1089 (12.8296, -4.3) -> (12.9125, -4.287)
  line L1090 (12.9925, -4.2654) -> (12.9125, -4.287)
  line L1091 (12.9125, -4.287) -> (12.9925, -4.2654)
  line L1092 (13.0711, -4.2358) -> (12.9925, -4.2654)
  line L1093 (12.9925, -4.2654) -> (13.0711, -4.2358)
  line L1094 (13.1237, -4.2099) -> (13.0711, -4.2358)
  line L1095 (13.0711, -4.2358) -> (13.1237, -4.2099)
  line L1096 (13.1944, -4.1659) -> (13.1237, -4.2099)
  line L1097 (13.1237, -4.2099) -> (13.1944, -4.1659)
  line L1098 (13.2593, -4.1147) -> (13.1944, -4.1659)
  line L1099 (13.1944, -4.1659) -> (13.2593, -4.1147)
  line L1100 (13.3169, -4.0549) -> (13.2593, -4.1147)
  line L1101 (13.2593, -4.1147) -> (13.3169, -4.0549)
  line L1102 (13.3681, -3.9878) -> (13.3169, -4.0549)
  line L1103 (13.3169, -4.0549) -> (13.3681, -3.9878)
  line L1104 (13.3999, -3.9352) -> (13.3681, -3.9878)
  line L1105 (13.3681, -3.9878) -> (13.3999, -3.9352)
  line L1106 (13.428, -3.8804) -> (13.3999, -3.9352)
  line L1107 (13.3999, -3.9352) -> (13.428, -3.8804)
  line L1108 (13.4554, -3.817) -> (13.428, -3.8804)
  line L1109 (13.428, -3.8804) -> (13.4554, -3.817)
  line L1110 (13.4813, -3.7456) -> (13.4554, -3.817)
  line L1111 (13.4554, -3.817) -> (13.4813, -3.7456)
  line L1112 (13.5073, -3.6663) -> (13.4813, -3.7456)
  line L1113 (13.4813, -3.7456) -> (13.5073, -3.6663)
  line L1114 (13.5318, -3.5783) -> (13.5073, -3.6663)
  line L1115 (13.5073, -3.6663) -> (13.5318, -3.5783)
  line L1116 (13.5556, -3.4817) -> (13.5318, -3.5783)
  line L1117 (13.5318, -3.5783) -> (13.5556, -3.4817)
  line L1118 (13.5794, -3.3772) -> (13.5556, -3.4817)
  line L1119 (13.5556, -3.4817) -> (13.5794, -3.3772)
  line L1120 (13.5837, -3.3548) -> (13.5794, -3.3772)
  line L1121 (13.5794, -3.3772) -> (13.5837, -3.3548)
  line L1122 (13.8908, -1.887) -> (13.5837, -3.3548)
  line L1123 (13.5837, -3.3548) -> (13.8908, -1.887)
  line L1124 (14.247, -1.887) -> (13.8908, -1.887)
  line L1125 (13.8908, -1.887) -> (14.247, -1.887)
  line L1126 (13.9218, -3.4514) -> (14.247, -1.887)
  line L1127 (14.247, -1.887) -> (13.9218, -3.4514)
  line L1128 (13.9002, -3.5495) -> (13.9218, -3.4514)
  line L1129 (13.9218, -3.4514) -> (13.9002, -3.5495)
  line L1130 (13.8764, -3.6418) -> (13.9002, -3.5495)
  line L1131 (13.9002, -3.5495) -> (13.8764, -3.6418)
  line L1132 (13.8512, -3.7297) -> (13.8764, -3.6418)
  line L1133 (13.8764, -3.6418) -> (13.8512, -3.7297)
  line L1134 (13.8245, -3.8119) -> (13.8512, -3.7297)
  line L1135 (13.8512, -3.7297) -> (13.8245, -3.8119)
  line L1136 (13.7957, -3.8891) -> (13.8245, -3.8119)
  line L1137 (13.8245, -3.8119) -> (13.7957, -3.8891)
  line L1138 (13.7654, -3.9604) -> (13.7957, -3.8891)
  line L1139 (13.7957, -3.8891) -> (13.7654, -3.9604)
  line L1140 (13.7337, -4.0268) -> (13.7654, -3.9604)
  line L1141 (13.7654, -3.9604) -> (13.7337, -4.0268)
  line L1142 (13.7019, -4.0837) -> (13.7337, -4.0268)
  line L1143 (13.7337, -4.0268) -> (13.7019, -4.0837)
  line L1144 (13.6565, -4.1551) -> (13.7019, -4.0837)
  line L1145 (13.7019, -4.0837) -> (13.6565, -4.1551)
  line L1146 (13.606, -4.2214) -> (13.6565, -4.1551)
  line L1147 (13.6565, -4.1551) -> (13.606, -4.2214)
  line L1148 (13.5513, -4.2834) -> (13.606, -4.2214)
  line L1149 (13.606, -4.2214) -> (13.5513, -4.2834)
  line L1150 (13.49, -4.3404) -> (13.5513, -4.2834)
  line L1151 (13.5513, -4.2834) -> (13.49, -4.3404)
  line L1152 (13.4244, -4.393) -> (13.49, -4.3404)
  line L1153 (13.49, -4.3404) -> (13.4244, -4.393)
  line L1154 (13.3537, -4.4406) -> (13.4244, -4.393)
  line L1155 (13.4244, -4.393) -> (13.3537, -4.4406)
  line L1156 (13.3234, -4.4586) -> (13.3537, -4.4406)
  line L1157 (13.3537, -4.4406) -> (13.3234, -4.4586)
  line L1158 (13.2528, -4.4968) -> (13.3234, -4.4586)
  line L1159 (13.3234, -4.4586) -> (13.2528, -4.4968)
  line L1160 (13.1785, -4.5285) -> (13.2528, -4.4968)
  line L1161 (13.2528, -4.4968) -> (13.1785, -4.5285)
  line L1162 (13.1014, -4.5545) -> (13.1785, -4.5285)
  line L1163 (13.1785, -4.5285) -> (13.1014, -4.5545)
  line L1164 (13.0206, -4.5747) -> (13.1014, -4.5545)
  line L1165 (13.1014, -4.5545) -> (13.0206, -4.5747)
  line L1166 (12.937, -4.5891) -> (13.0206, -4.5747)
  line L1167 (13.0206, -4.5747) -> (12.937, -4.5891)
  line L1168 (12.8498, -4.5978) -> (12.937, -4.5891)
  line L1169 (12.937, -4.5891) -> (12.8498, -4.5978)
  line L1170 (12.7618, -4.6006) -> (12.8498, -4.5978)
  line L1171 (12.8498, -4.5978) -> (12.7618, -4.6006)
  line L1172 (12.6688, -4.5985) -> (12.7618, -4.6006)
  line L1173 (12.7618, -4.6006) -> (12.6688, -4.5985)
  line L1174 (12.5794, -4.5906) -> (12.6688, -4.5985)
  line L1175 (12.6688, -4.5985) -> (12.5794, -4.5906)
  line L1176 (12.4951, -4.5783) -> (12.5794, -4.5906)
  line L1177 (12.5794, -4.5906) -> (12.4951, -4.5783)
  line L1178 (12.4136, -4.561) -> (12.4951, -4.5783)
  line L1179 (12.4951, -4.5783) -> (12.4136, -4.561)
  line L1180 (12.3372, -4.5386) -> (12.4136, -4.561)
  line L1181 (12.4136, -4.561) -> (12.3372, -4.5386)
  line L1182 (12.2644, -4.5112) -> (12.3372, -4.5386)
  line L1183 (12.3372, -4.5386) -> (12.2644, -4.5112)
  line L1184 (12.2406, -4.5004) -> (12.2644, -4.5112)
  line L1185 (12.2644, -4.5112) -> (12.2406, -4.5004)
  line L1186 (12.1591, -4.4593) -> (12.2406, -4.5004)
  line L1187 (12.2406, -4.5004) -> (12.1591, -4.4593)
  line L1188 (12.087, -4.4125) -> (12.1591, -4.4593)
  line L1189 (12.1591, -4.4593) -> (12.087, -4.4125)
  line L1190 (12.0228, -4.3606) -> (12.087, -4.4125)
  line L1191 (12.087, -4.4125) -> (12.0228, -4.3606)
  line L1192 (11.9666, -4.3022) -> (12.0228, -4.3606)
  line L1193 (12.0228, -4.3606) -> (11.9666, -4.3022)
  line L1194 (11.919, -4.2387) -> (11.9666, -4.3022)
  line L1195 (11.9666, -4.3022) -> (11.919, -4.2387)
  line L1196 (11.9096, -4.2243) -> (11.919, -4.2387)
  line L1197 (11.919, -4.2387) -> (11.9096, -4.2243)
  line L1198 (11.8693, -4.1515) -> (11.9096, -4.2243)
  line L1199 (11.9096, -4.2243) -> (11.8693, -4.1515)
  line L1200 (11.8383, -4.0758) -> (11.8693, -4.1515)
  line L1201 (11.8693, -4.1515) -> (11.8383, -4.0758)
  line L1202 (11.8166, -3.9958) -> (11.8383, -4.0758)
  line L1203 (11.8383, -4.0758) -> (11.8166, -3.9958)
  line L1204 (11.8029, -3.9121) -> (11.8166, -3.9958)
  line L1205 (11.8166, -3.9958) -> (11.8029, -3.9121)
  line L1206 (11.7986, -3.8249) -> (11.8029, -3.9121)
  line L1207 (11.8029, -3.9121) -> (11.7986, -3.8249)
  line L1208 (11.7986, -3.8242) -> (11.7986, -3.8249)
  line L1209 (11.7986, -3.8249) -> (11.7986, -3.8242)
  line L1210 (11.8008, -3.7694) -> (11.7986, -3.8242)
  line L1211 (11.7986, -3.8242) -> (11.8008, -3.7694)
  line L1212 (11.8073, -3.7023) -> (11.8008, -3.7694)
  line L1213 (11.8008, -3.7694) -> (11.8073, -3.7023)
  line L1214 (11.8188, -3.623) -> (11.8073, -3.7023)
  line L1215 (11.8073, -3.7023) -> (11.8188, -3.623)
  line L1216 (11.8347, -3.5315) -> (11.8188, -3.623)
  line L1217 (11.8188, -3.623) -> (11.8347, -3.5315)
  line L1218 (11.8548, -3.4276) -> (11.8347, -3.5315)
  line L1219 (11.8347, -3.5315) -> (11.8548, -3.4276)
  line L1220 (11.8729, -3.3419) -> (11.8548, -3.4276)
  line L1221 (11.8548, -3.4276) -> (11.8729, -3.3419)
  line L1222 (12.1764, -1.887) -> (11.8729, -3.3419)
  line L1223 (11.8729, -3.3419) -> (12.1764, -1.887)
  line L1224 (12.5333, -1.887) -> (12.1764, -1.887)
  line L1225 (12.1764, -1.887) -> (12.5333, -1.887)
  line L1226 (5.3453, -4.3663) -> (5.4174, -4.3274)
  line L1227 (5.4174, -4.3274) -> (5.3453, -4.3663)
  line L1228 (5.2704, -4.4024) -> (5.3453, -4.3663)
  line L1229 (5.3453, -4.3663) -> (5.2704, -4.4024)
  line L1230 (5.1925, -4.437) -> (5.2704, -4.4024)
  line L1231 (5.2704, -4.4024) -> (5.1925, -4.437)
  line L1232 (5.1118, -4.4687) -> (5.1925, -4.437)
  line L1233 (5.1925, -4.437) -> (5.1118, -4.4687)
  line L1234 (5.0281, -4.4975) -> (5.1118, -4.4687)
  line L1235 (5.1118, -4.4687) -> (5.0281, -4.4975)
  line L1236 (4.9849, -4.5112) -> (5.0281, -4.4975)
  line L1237 (5.0281, -4.4975) -> (4.9849, -4.5112)
  line L1238 (4.9005, -4.5358) -> (4.9849, -4.5112)
  line L1239 (4.9849, -4.5112) -> (4.9005, -4.5358)
  line L1240 (4.8162, -4.5559) -> (4.9005, -4.5358)
  line L1241 (4.9005, -4.5358) -> (4.8162, -4.5559)
  line L1242 (4.7325, -4.5725) -> (4.8162, -4.5559)
  line L1243 (4.8162, -4.5559) -> (4.7325, -4.5725)
  line L1244 (4.6489, -4.5848) -> (4.7325, -4.5725)
  line L1245 (4.7325, -4.5725) -> (4.6489, -4.5848)
  line L1246 (4.566, -4.5934) -> (4.6489, -4.5848)
  line L1247 (4.6489, -4.5848) -> (4.566, -4.5934)
  line L1248 (4.4838, -4.5978) -> (4.566, -4.5934)
  line L1249 (4.566, -4.5934) -> (4.4838, -4.5978)
  line L1250 (4.4305, -4.5985) -> (4.4838, -4.5978)
  line L1251 (4.4838, -4.5978) -> (4.4305, -4.5985)
  line L1252 (4.3338, -4.5963) -> (4.4305, -4.5985)
  line L1253 (4.4305, -4.5985) -> (4.3338, -4.5963)
  line L1254 (4.2416, -4.5884) -> (4.3338, -4.5963)
  line L1255 (4.3338, -4.5963) -> (4.2416, -4.5884)
  line L1256 (4.1529, -4.5761) -> (4.2416, -4.5884)
  line L1257 (4.2416, -4.5884) -> (4.1529, -4.5761)
  line L1258 (4.0693, -4.5581) -> (4.1529, -4.5761)
  line L1259 (4.1529, -4.5761) -> (4.0693, -4.5581)
  line L1260 (3.9899, -4.5358) -> (4.0693, -4.5581)
  line L1261 (4.0693, -4.5581) -> (3.9899, -4.5358)
  line L1262 (3.9142, -4.5076) -> (3.9899, -4.5358)
  line L1263 (3.9899, -4.5358) -> (3.9142, -4.5076)
  line L1264 (3.8429, -4.4752) -> (3.9142, -4.5076)
  line L1265 (3.9142, -4.5076) -> (3.8429, -4.4752)
  line L1266 (3.7765, -4.437) -> (3.8429, -4.4752)
  line L1267 (3.8429, -4.4752) -> (3.7765, -4.437)
  line L1268 (3.7138, -4.3937) -> (3.7765, -4.437)
  line L1269 (3.7765, -4.437) -> (3.7138, -4.3937)
  line L1270 (3.6554, -4.3461) -> (3.7138, -4.3937)
  line L1271 (3.7138, -4.3937) -> (3.6554, -4.3461)
  line L1272 (3.6006, -4.2928) -> (3.6554, -4.3461)
  line L1273 (3.6554, -4.3461) -> (3.6006, -4.2928)
  line L1274 (3.561, -4.2481) -> (3.6006, -4.2928)
  line L1275 (3.6006, -4.2928) -> (3.561, -4.2481)
  line L1276 (3.5141, -4.1854) -> (3.561, -4.2481)
  line L1277 (3.561, -4.2481) -> (3.5141, -4.1854)
  line L1278 (3.4723, -4.119) -> (3.5141, -4.1854)
  line L1279 (3.5141, -4.1854) -> (3.4723, -4.119)
  line L1280 (3.4355, -4.0498) -> (3.4723, -4.119)
  line L1281 (3.4723, -4.119) -> (3.4355, -4.0498)
  line L1282 (3.4038, -3.977) -> (3.4355, -4.0498)
  line L1283 (3.4355, -4.0498) -> (3.4038, -3.977)
  line L1284 (3.3771, -3.9006) -> (3.4038, -3.977)
  line L1285 (3.4038, -3.977) -> (3.3771, -3.9006)
  line L1286 (3.3555, -3.8198) -> (3.3771, -3.9006)
  line L1287 (3.3771, -3.9006) -> (3.3555, -3.8198)
  line L1288 (3.3389, -3.7362) -> (3.3555, -3.8198)
  line L1289 (3.3555, -3.8198) -> (3.3389, -3.7362)
  line L1290 (3.3274, -3.649) -> (3.3389, -3.7362)
  line L1291 (3.3389, -3.7362) -> (3.3274, -3.649)
  line L1292 (3.3209, -3.5589) -> (3.3274, -3.649)
  line L1293 (3.3274, -3.649) -> (3.3209, -3.5589)
  line L1294 (3.3195, -3.4853) -> (3.3209, -3.5589)
  line L1295 (3.3209, -3.5589) -> (3.3195, -3.4853)
  line L1296 (3.3216, -3.3974) -> (3.3195, -3.4853)
  line L1297 (3.3195, -3.4853) -> (3.3216, -3.3974)
  line L1298 (3.3267, -3.3109) -> (3.3216, -3.3974)
  line L1299 (3.3216, -3.3974) -> (3.3267, -3.3109)
  line L1300 (3.336, -3.2258) -> (3.3267, -3.3109)
  line L1301 (3.3267, -3.3109) -> (3.336, -3.2258)
  line L1302 (3.349, -3.1414) -> (3.336, -3.2258)
  line L1303 (3.336, -3.2258) -> (3.349, -3.1414)
  line L1304 (3.3649, -3.0592) -> (3.349, -3.1414)
  line L1305 (3.349, -3.1414) -> (3.3649, -3.0592)
  line L1306 (3.3851, -2.9785) -> (3.3649, -3.0592)
  line L1307 (3.3649, -3.0592) -> (3.3851, -2.9785)
  line L1308 (3.4089, -2.8992) -> (3.3851, -2.9785)
  line L1309 (3.3851, -2.9785) -> (3.4089, -2.8992)
  line L1310 (3.4363, -2.8213) -> (3.4089, -2.8992)
  line L1311 (3.4089, -2.8992) -> (3.4363, -2.8213)
  line L1312 (3.4673, -2.7449) -> (3.4363, -2.8213)
  line L1313 (3.4363, -2.8213) -> (3.4673, -2.7449)
  line L1314 (3.5019, -2.6699) -> (3.4673, -2.7449)
  line L1315 (3.4673, -2.7449) -> (3.5019, -2.6699)
  line L1316 (3.5321, -2.6108) -> (3.5019, -2.6699)
  line L1317 (3.5019, -2.6699) -> (3.5321, -2.6108)
  line L1318 (3.5776, -2.5308) -> (3.5321, -2.6108)
  line L1319 (3.5321, -2.6108) -> (3.5776, -2.5308)
  line L1320 (3.6259, -2.4551) -> (3.5776, -2.5308)
  line L1321 (3.5776, -2.5308) -> (3.6259, -2.4551)
  line L1322 (3.6763, -2.3837) -> (3.6259, -2.4551)
  line L1323 (3.6259, -2.4551) -> (3.6763, -2.3837)
  line L1324 (3.729, -2.3167) -> (3.6763, -2.3837)
  line L1325 (3.6763, -2.3837) -> (3.729, -2.3167)
  line L1326 (3.7845, -2.2547) -> (3.729, -2.3167)
  line L1327 (3.729, -2.3167) -> (3.7845, -2.2547)
  line L1328 (3.8429, -2.197) -> (3.7845, -2.2547)
  line L1329 (3.7845, -2.2547) -> (3.8429, -2.197)
  line L1330 (3.9027, -2.1436) -> (3.8429, -2.197)
  line L1331 (3.8429, -2.197) -> (3.9027, -2.1436)
  line L1332 (3.9662, -2.0946) -> (3.9027, -2.1436)
  line L1333 (3.9027, -2.1436) -> (3.9662, -2.0946)
  line L1334 (4.031, -2.0499) -> (3.9662, -2.0946)
  line L1335 (3.9662, -2.0946) -> (4.031, -2.0499)
  line L1336 (4.0664, -2.029) -> (4.031, -2.0499)
  line L1337 (4.031, -2.0499) -> (4.0664, -2.029)
  line L1338 (4.1399, -1.9893) -> (4.0664, -2.029)
  line L1339 (4.0664, -2.029) -> (4.1399, -1.9893)
  line L1340 (4.2149, -1.954) -> (4.1399, -1.9893)
  line L1341 (4.1399, -1.9893) -> (4.2149, -1.954)
  line L1342 (4.2913, -1.9237) -> (4.2149, -1.954)
  line L1343 (4.2149, -1.954) -> (4.2913, -1.9237)
  line L1344 (4.3706, -1.8985) -> (4.2913, -1.9237)
  line L1345 (4.2913, -1.9237) -> (4.3706, -1.8985)
  line L1346 (4.4506, -1.8776) -> (4.3706, -1.8985)
  line L1347 (4.3706, -1.8985) -> (4.4506, -1.8776)
  line L1348 (4.5328, -1.861) -> (4.4506, -1.8776)
  line L1349 (4.4506, -1.8776) -> (4.5328, -1.861)
  line L1350 (4.6172, -1.8502) -> (4.5328, -1.861)
  line L1351 (4.5328, -1.861) -> (4.6172, -1.8502)
  line L1352 (4.703, -1.843) -> (4.6172, -1.8502)
  line L1353 (4.6172, -1.8502) -> (4.703, -1.843)
  line L1354 (4.783, -1.8415) -> (4.703, -1.843)
  line L1355 (4.703, -1.843) -> (4.783, -1.8415)
  line L1356 (4.8731, -1.8437) -> (4.783, -1.8415)
  line L1357 (4.783, -1.8415) -> (4.8731, -1.8437)
  line L1358 (4.9604, -1.8516) -> (4.8731, -1.8437)
  line L1359 (4.8731, -1.8437) -> (4.9604, -1.8516)
  line L1360 (5.044, -1.8653) -> (4.9604, -1.8516)
  line L1361 (4.9604, -1.8516) -> (5.044, -1.8653)
  line L1362 (5.1247, -1.8841) -> (5.044, -1.8653)
  line L1363 (5.044, -1.8653) -> (5.1247, -1.8841)
  line L1364 (5.2026, -1.9079) -> (5.1247, -1.8841)
  line L1365 (5.1247, -1.8841) -> (5.2026, -1.9079)
  line L1366 (5.2776, -1.9367) -> (5.2026, -1.9079)
  line L1367 (5.2026, -1.9079) -> (5.2776, -1.9367)
  line L1368 (5.292, -1.9432) -> (5.2776, -1.9367)
  line L1369 (5.2776, -1.9367) -> (5.292, -1.9432)
  line L1370 (5.3735, -1.985) -> (5.292, -1.9432)
  line L1371 (5.292, -1.9432) -> (5.3735, -1.985)
  line L1372 (5.447, -2.0312) -> (5.3735, -1.985)
  line L1373 (5.3735, -1.985) -> (5.447, -2.0312)
  line L1374 (5.5133, -2.0816) -> (5.447, -2.0312)
  line L1375 (5.447, -2.0312) -> (5.5133, -2.0816)
  line L1376 (5.5717, -2.1379) -> (5.5133, -2.0816)
  line L1377 (5.5133, -2.0816) -> (5.5717, -2.1379)
  line L1378 (4.6878, -2.1415) -> (4.7722, -2.1379)
  line L1379 (4.7722, -2.1379) -> (4.6878, -2.1415)
  line L1380 (4.6049, -2.1516) -> (4.6878, -2.1415)
  line L1381 (4.6878, -2.1415) -> (4.6049, -2.1516)
  line L1382 (4.5242, -2.1681) -> (4.6049, -2.1516)
  line L1383 (4.6049, -2.1516) -> (4.5242, -2.1681)
  line L1384 (4.4449, -2.1919) -> (4.5242, -2.1681)
  line L1385 (4.5242, -2.1681) -> (4.4449, -2.1919)
  line L1386 (4.367, -2.2229) -> (4.4449, -2.1919)
  line L1387 (4.4449, -2.1919) -> (4.367, -2.2229)
  line L1388 (4.2906, -2.2604) -> (4.367, -2.2229)
  line L1389 (4.367, -2.2229) -> (4.2906, -2.2604)
  line L1390 (4.2322, -2.2943) -> (4.2906, -2.2604)
  line L1391 (4.2906, -2.2604) -> (4.2322, -2.2943)
  line L1392 (4.1673, -2.339) -> (4.2322, -2.2943)
  line L1393 (4.2322, -2.2943) -> (4.1673, -2.339)
  line L1394 (4.1053, -2.3902) -> (4.1673, -2.339)
  line L1395 (4.1673, -2.339) -> (4.1053, -2.3902)
  line L1396 (4.0476, -2.4464) -> (4.1053, -2.3902)
  line L1397 (4.1053, -2.3902) -> (4.0476, -2.4464)
  line L1398 (3.9936, -2.5084) -> (4.0476, -2.4464)
  line L1399 (4.0476, -2.4464) -> (3.9936, -2.5084)
  line L1400 (3.9431, -2.5755) -> (3.9936, -2.5084)
  line L1401 (3.9936, -2.5084) -> (3.9431, -2.5755)
  line L1402 (3.8955, -2.649) -> (3.9431, -2.5755)
  line L1403 (3.9431, -2.5755) -> (3.8955, -2.649)
  line L1404 (3.8522, -2.7276) -> (3.8955, -2.649)
  line L1405 (3.8955, -2.649) -> (3.8522, -2.7276)
  line L1406 (3.8321, -2.7687) -> (3.8522, -2.7276)
  line L1407 (3.8522, -2.7276) -> (3.8321, -2.7687)
  line L1408 (3.7996, -2.8422) -> (3.8321, -2.7687)
  line L1409 (3.8321, -2.7687) -> (3.7996, -2.8422)